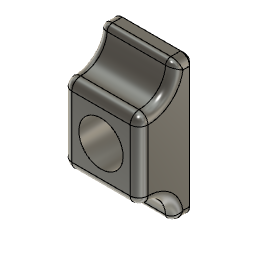
[a]_belt_clamp_x2 (Autodesk Fusion 360 design; units mm, degrees)
Autodesk Fusion 360 part; units mm, degrees
sketch "Sketch1" plane through (0, 0, 0) normal (0, 1, 0) x (1, 0, 0) in component "[a]_belt_clamp_x2"
  line L0 (4.25, 7.875) -> (-4.25, 7.875)
  line L1 (-4.25, 7.875) -> (-4.25, -7.875)
  line L2 (-4.25, -7.875) -> (4.25, -7.875)
  line L3 (4.25, -7.875) -> (4.25, 7.875)
  line L4 (4.25, 7.875) -> (-4.25, -7.875) construction
  line L5 (-4.25, 7.875) -> (4.25, -7.875) construction
  dimension "d1" = 8.5
  dimension "d2" = 15.75
  constraint horizontal L0
  constraint perpendicular L0 L1
  constraint parallel L0 L2
  constraint parallel L1 L3
  constraint coincident L4 origin
  constraint coincident L5 origin
  measures "d1" distance of L1.end L2.end
  measures "d2" distance of L0.end L1.end
sketch "Sketch2" plane through (0, 0, 0) normal (1, 0, 0) x (0, 1, 0) in component "[a]_belt_clamp_x2"
  line L0 (2.55, 7.875) -> (-3.55, 7.875)
  line L1 (-3.55, 7.875) -> (-3.55, -7.875)
  line L2 (-3.55, -7.875) -> (2.55, -7.875)
  line L3 (2.55, -7.875) -> (2.55, 7.875)
  line L4 (2.55, 7.875) -> (-3.55, -7.875) construction
  line L5 (-3.55, 7.875) -> (2.55, -7.875) construction
  line L6 (-3.55, 4.475) -> (-2.55, 4.475)
  line L7 (0.45, 7.475) -> (0.45, 7.875)
  arc A0 (-2.55, 4.475) -> (0.45, 7.475) centre (-2.55, 7.475) ccw
  line L8 (0, 0) -> (-7.5, 0) construction
  line L9 (-3.55, -4.475) -> (-2.55, -4.475)
  arc A1 (0.45, -7.475) -> (-2.55, -4.475) centre (-2.55, -7.475) ccw
  line L10 (0.45, -7.475) -> (0.45, -7.875)
  point P0 (-0.5, 0)
  dimension "d8" = 6.1
  dimension "d9" = 15.75
  dimension "d10" = 3
  dimension "d11" = 3.4
  dimension "d12" = 3
  dimension "d13" = 1
  constraint horizontal L0
  constraint perpendicular L0 L1
  constraint parallel L0 L2
  constraint parallel L1 L3
  constraint coincident L4 P0
  constraint coincident L5 P0
  constraint coincident L1 L6.start
  constraint perpendicular L1 L6
  constraint coincident L0 L7.end
  constraint perpendicular L0 L7
  constraint tangent L6 A0
  constraint coincident L8.start origin
  constraint perpendicular L1 L8
  constraint symmetric L6.start L8 L9.start
  constraint symmetric L6.end L8 L9.end
  constraint symmetric L7.start L8 A1.start
  constraint symmetric L7.end L8 L10.end
  constraint symmetric A0 L8 A1
  measures "d8" distance of L1.end L2.end
  measures "d9" distance of L0.end L1.end
  measures "d10" vertical distance of L6.end L7.start
  measures "d11" distance of L0 L6.end
  measures "d12" horizontal distance of L6.end L7.start
  measures "d13" distance of L1 L6.end
extrude "Extrude2" add sketch "Sketch2" along normal mid plane 8.6 contours L0 L1 L2 L3 L6 L7 A0 L9 A1 L10 in component "[a]_belt_clamp_x2"
fillet "Fillet1" radius 0.6 2 edges at (0, 0.45, 7.875) (0, 0.45, -7.875) in component "[a]_belt_clamp_x2"
fillet "Fillet2" radius 1 20 edges at (-4.3, -3.05, 4.475) (-4.3, -0.4884, 5.2956) (-4.3, 0.6321, 7.7109) (-4.3, 1.7972, 7.875) (4.3, -3.05, 4.475) (4.3, -0.4884, 5.2956) (4.3, 0.6321, 7.7109) (4.3, 1.7972, 7.875) (-4.3, 1.7972, -7.875) (-4.3, 0.6321, -7.7109) (-4.3, -0.4884, -5.2956) (-4.3, -3.05, -4.475) (4.3, -3.05, -4.475) (4.3, -0.4884, -5.2956) (4.3, 0.6321, -7.7109) (4.3, 1.7972, -7.875) (0, -3.55, 4.475) (-4.3, -3.55, 0) (0, -3.55, -4.475) (4.3, -3.55, 0) in component "[a]_belt_clamp_x2"
hole "Hole1" at (0, -3.55, 0) direction (0, 1, 0) diameter 5 depth 4 tip angle 180 in component "[a]_belt_clamp_x2"
hole "Hole2" at (0, 0.45, 0) direction (0, 1, 0) diameter 3.4 end through all in component "[a]_belt_clamp_x2"
chamfer "Chamfer1" distance 0.4 angle 45 9 edges at (4.0071, 2.55, 7.5821) (0, 2.55, 7.875) (-4.0071, 2.55, 7.5821) (-4.3, 2.55, 0) (-4.0071, 2.55, -7.5821) (0, 2.55, -7.875) (4.0071, 2.55, -7.5821) (4.3, 2.55, 0) (-0.6147, 2.55, 1.585) in component "[a]_belt_clamp_x2"
component "[a]_belt_clamp_x2" placed x (1, 0, 0) y (0, 1, 0) z (0, 0, 1) at (0, 0, 0)
equation "d2 = ab_belt_width * 2 + 3.75 mm"
equation "ab_belt_width = 6 mm"
equation "d9 = ab_belt_width * 2 + 3.75 mm"
equation "d21 = ( 2.5 * 2 ) * 1 mm"
equation "d24 = ( 1.7 * 2 ) * 1 mm"
